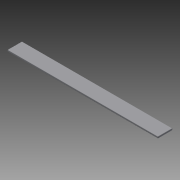
# Autodesk Inventor part: CeramicModel
Saved by Autodesk Inventor 2015 SP1 (Build 190203100, 203)
## iProperties
Created: 2015-10-16
Part Number: CeramicModel
Material: Generic
Document SubType Name: Modeling
Designer: I Rabey
Density: 1 g/cm^3
Appearance: Default
Author: I Rabey
Autodesk Inventor part; units mm, degrees
ref_plane "YZ Plane" through (0, 0, 0) normal (1, 0, 0) x (0, 1, 0)
ref_plane "XZ Plane" through (0, 0, 0) normal (0, 1, 0) x (-1, 0, 0)
ref_plane "XY Plane" through (0, 0, 0) normal (0, 0, 1) x (1, 0, 0)
sketch "Sketch1" plane through (0, 0, 0) normal (1, 0, 0) x (0, 1, 0)
  line L0 (-3, 40) -> (3, 40)
  line L1 (5, 38) -> (5, -38)
  line L2 (3, -40) -> (-3, -40)
  line L3 (-5, -38) -> (-5, 38)
  line L4 (-5, 40) -> (5, -40) construction
  line L5 (5, 40) -> (-5, -40) construction
  arc A0 (5, 38) -> (3, 40) centre (3, 38) ccw
  arc A1 (-3, 40) -> (-5, 38) centre (-3, 38) ccw
  arc A2 (3, -40) -> (5, -38) centre (3, -38) ccw
  arc A3 (-5, -38) -> (-3, -40) centre (-3, -38) ccw
  point P0 (0, 0)
  dimension "d0" = 10
  dimension "d1" = 80
  dimension "d2" = 2
  constraints: 12 end point, 8 point on circle, 8 point on line, 8 tangent, 4 centre point, 3 equal radius, 2 midpoint, 2 parallel, 1 horizontal, 1 perpendicular
  measures "d0" distance of L4.end L5.end
  measures "d1" distance of L5.start L4.end
  measures "d2" radius of A0
extrude "Extrusion1" add sketch "Sketch1" along normal blind 417.5 and the other way blind 417.5
fillet "Fillet1" radius 2 8 edges at (417.5, 4.4142, 39.4142) (417.5, 0, 40) (417.5, -4.4142, 39.4142) (417.5, -5, 0) (417.5, -4.4142, -39.4142) (417.5, 0, -40) (417.5, 4.4142, -39.4142) (417.5, 5, 0)
fillet "Fillet2" radius 2 8 edges at (-417.5, 4.4142, -39.4142) (-417.5, 0, -40) (-417.5, -4.4142, -39.4142) (-417.5, -5, 0) (-417.5, -4.4142, 39.4142) (-417.5, 0, 40) (-417.5, 4.4142, 39.4142) (-417.5, 5, 0)
body "Solid1"
